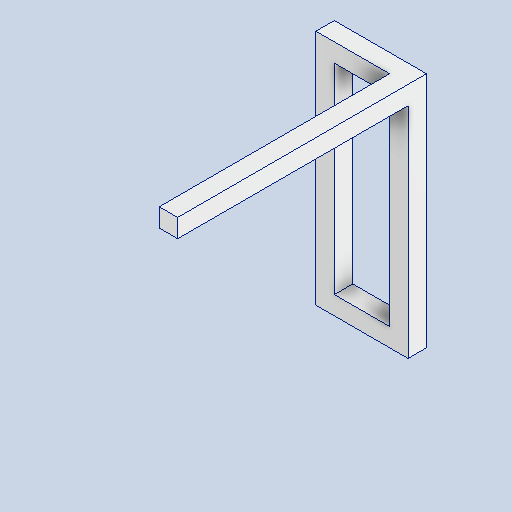
# Autodesk Inventor part: FrameSide
Saved by Autodesk Inventor 2025 (Build 290162010, 162A)
## iProperties
Created: 2024-11-18
Part Number: FrameSide
Material: Aluminium 6061, Frame
Document SubType Name: Modeling
Designer: Admin
Density: 2.7 g/cm^3
Appearance: Aluminium - flach(2)
Mass: 7646.4 g
Surface Area: 2832 cm^2
Volume: 2832 cm^3
Author: Admin
Autodesk Inventor part; units mm, degrees
ref_plane "YZ Plane" through (0, 0, 0) normal (1, 0, 0) x (0, 1, 0)
ref_plane "XZ Plane" through (0, 0, 0) normal (0, 1, 0) x (-1, 0, 0)
ref_plane "XY Plane" through (0, 0, 0) normal (0, 0, 1) x (1, 0, 0)
sketch "Skizze1" plane through (0, 0, 0) normal (0, 0, 1) x (1, 0, 0)
  line L0 (0, 0) -> (32, 0) construction
  line L1 (-84, 5) -> (-84, -35)
  line L2 (-84, -35) -> (116, -35)
  line L3 (116, -35) -> (116, 5)
  line L4 (-84, 5) -> (116, 5)
  line L5 (0, 0) -> (-84, 0) construction
  line L6 (32, 0) -> (116, 0) construction
  point P0 (16, 5)
  dimension "d0" = 200
  dimension "d1" = 40
  dimension "d2" = 5
  constraints: 12 end point, 3 perpendicular, 3 point on line, 2 horizontal, 1 collinear, 1 midpoint
  measures "d0" distance of L1.end L2.end
  measures "d1" distance of L1.start L1.end
  measures "d2" distance from line of point (16, 5) L0
extrude "Extrusion1" add sketch "Skizze1" along normal blind 40
sketch "Skizze2" plane through (0, 0, 40) normal (0, 0, 1) x (1, 0, 0)
  line L0 (116, -35) -> (116, 5) projected
  line L1 (-84, 5) -> (-84, -35) projected
  line L2 (116, -35) -> (76, -35)
  line L3 (76, -35) -> (76, 5)
  line L4 (76, 5) -> (116, 5)
  line L5 (-84, -35) -> (-44, -35)
  line L6 (-44, -35) -> (-44, 5)
  line L7 (-44, 5) -> (-84, 5)
  point P0 (0, 0)
  constraints: 12 end point, 6 perpendicular, 1 parallel, 1 vertical
extrude "Extrusion2" add sketch "Skizze2" along normal blind 475
sketch "Skizze3" plane through (0, 0, 515) normal (0, 0, 1) x (1, 0, 0)
  line L0 (116, -35) -> (116, 5) projected
  line L1 (-84, 5) -> (-84, -35) projected
  line L2 (76, -35) -> (116, -35) projected
  line L3 (116, -35) -> (-84, -35)
  line L4 (116, 5) -> (-84, 5)
  point P0 (0, 0)
  constraints: 4 end point, 1 collinear, 1 horizontal
extrude "Extrusion3" add sketch "Skizze3" against normal blind 40
ref_plane "Arbeitsebene1" through (34.1, -565, 450) normal (0, 1, 0) x (0, 0, 1)
sketch "Skizze4" plane through (-84, -35, 0) normal (0, -1, 0) x (1, 0, 0)
  line L0 (136.45, -16.1) -> (139.75, -16.1) construction
  line L1 (138.1, -16.1) -> (138.1, 515) construction
  line L2 (0, 515) -> (200, 515) construction
  line L3 (160, 515) -> (200, 515)
  line L4 (200, 515) -> (200, 475)
  line L5 (200, 475) -> (160, 475)
  line L6 (160, 475) -> (160, 515)
  line L7 (200, 0) -> (200, 515) projected
  point P0 (84, 0)
  dimension "d10" = 40
  dimension "d26" = 40
  dimension "d27" = 0
  constraints: 10 end point, 2 parallel, 2 point on line, 1 horizontal, 1 midpoint, 1 perpendicular, 1 vertical
  measures "d10" distance of L3.end L4.end
  measures "d26" distance between parallel lines of L4 L6
  measures "d27" distance between parallel lines of L7 L4
extrude "Extrusion4" add sketch "Skizze4" along normal blind 500
equation "\"d5\" = höheFrame"
equation "\"höheFrame\" = 475"
